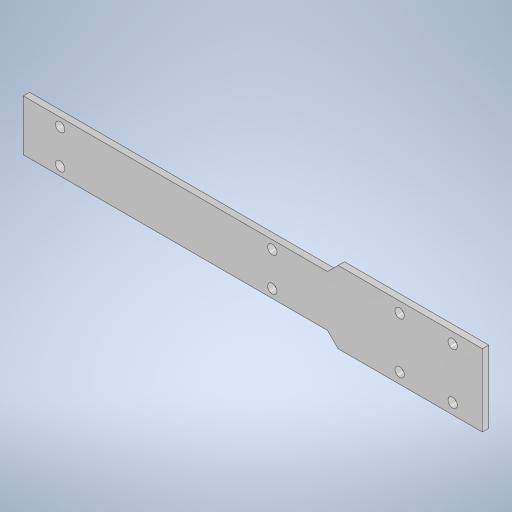
# Autodesk Inventor part: slider_plate
Saved by Autodesk Inventor 2024 (Build 280153000, 153)
## iProperties
Created: 2025-06-12
Part Number: slider_plate
Material: アルミニウム
Document SubType Name: Modeling
Designer: 1412z
Density: 2.7 g/cm^3
Appearance: アルミニウム - つや出し
Author: 1412z
Autodesk Inventor part; units mm, degrees
ref_plane "YZ Plane" through (0, 0, 0) normal (1, 0, 0) x (0, 1, 0)
ref_plane "XZ Plane" through (0, 0, 0) normal (0, 1, 0) x (-1, 0, 0)
ref_plane "XY Plane" through (0, 0, 0) normal (0, 0, 1) x (1, 0, 0)
sketch "スケッチ1" plane through (0, 0, 0) normal (0, 0, 1) x (1, 0, 0)
  line L0 (0, 0) -> (-94.2, 0)
  line L1 (-94.2, 0) -> (-94.2, -12)
  line L2 (-94.2, -12) -> (0, -12)
  line L3 (0, -12) -> (0, 0)
  circle A0 centre (-85.5, -2) radius 1.1
  circle A1 centre (-85.5, -10) radius 1.1
  circle A2 centre (-35.5, -10) radius 1.1
  circle A3 centre (-35.5, -2) radius 1.1
  dimension "d0" = 94.2
  dimension "d1" = 12
  dimension "d2" = 2.2
  dimension "d3" = 2.2
  dimension "d4" = 8.7
  dimension "d5" = 2.2
  dimension "d7" = 2.2
  dimension "d9" = 50
  dimension "d10" = 50
  constraints: 8 end point, 4 centre point, 2 parallel, 1 horizontal, 1 perpendicular
  measures "d0" distance of L2.end L1.end
  measures "d1" distance of L1.end L0.end
  measures "d2" diameter of A0
  measures "d3" diameter of A1
  measures "d4" distance from line of L1 A1.centre
  measures "d5" diameter of A2
  measures "d7" diameter of A3
  measures "d9" distance of A1.centre A2.centre
  measures "d10" distance of A0.centre A3.centre
extrude "押し出し1" add sketch "スケッチ1" along normal blind 1.5
sketch "スケッチ2" plane through (0, 0, 1.5) normal (0, 0, 1) x (1, 0, 0)
  line L0 (0, 2.5) -> (0, -14.5)
  line L1 (0, -14.5) -> (-20, -14.5)
  line L2 (-20, -14.5) -> (-22.5, -12)
  line L3 (-94.2, -12) -> (0, -12) projected
  line L4 (-22.5, -12) -> (-22.5, 0)
  line L5 (0, 0) -> (-94.2, 0) projected
  line L6 (0, 2.5) -> (-20, 2.5)
  line L7 (-20, 2.5) -> (-22.5, 0)
  dimension "d17" = 17
  dimension "d18" = 20
  dimension "d19" = 135
  constraints: 12 end point, 2 point on line, 1 horizontal, 1 parallel, 1 perpendicular, 1 vertical
  measures "d17" distance of L0.start L0.end
  measures "d18" distance of L0.end L1.end
  measures "d19" angle of L1 L2
extrude "押し出し2" add sketch "スケッチ2" against normal blind 1.5
sketch "スケッチ3" plane through (0, 0, 1.5) normal (0, 0, 1) x (1, 0, 0)
  circle A0 centre (-5.5, -12) radius 1.1
  circle A1 centre (-5.5, 0) radius 1.1
  point P0 (0, 0)
  dimension "d22" = 2.2
  dimension "d23" = 2.2
  constraints: 2 centre point
  measures "d22" diameter of A0
  measures "d23" diameter of A1
extrude "押し出し3" cut sketch "スケッチ3" against normal blind 1.5
sketch "スケッチ4" plane through (0, 0, 1.5) normal (0, 0, 1) x (1, 0, 0)
  line L0 (0, -14.5) -> (0, 2.5) projected
  line L1 (0, -6) -> (14, -6)
  line L2 (0, -6) -> (14, -6) construction
  line L3 (-20, -14.5) -> (0, -14.5) projected
  line L4 (0, -14.5) -> (14, -14.5)
  line L5 (14, -14.5) -> (14, 2.5)
  line L6 (-20, 2.5) -> (0, 2.5) projected
  line L7 (14, 2.5) -> (0, 2.5)
  line L8 (0, 2.5) -> (0, -14.5)
  circle A0 centre (7, -12) radius 1.1
  circle A1 centre (7, 0) radius 1.1
  point P0 (0, 0)
  dimension "d27" = 14
  dimension "d28" = 0
  dimension "d29" = 2.2
  dimension "d30" = 2.2
  constraints: 12 end point, 3 collinear, 3 horizontal, 2 centre point, 1 midpoint, 1 perpendicular
  measures "d27" distance of L1.start L1.end
  measures "d28" distance between parallel lines of L1 L2
  measures "d29" diameter of A0
  measures "d30" diameter of A1
extrude "押し出し4" add sketch "スケッチ4" against normal blind 1.5
